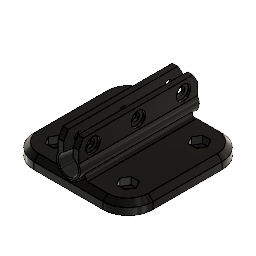
Thermometer Holder v4 (Autodesk Fusion 360 design; units mm, degrees)
Autodesk Fusion 360 part; units mm, degrees
sketch "Sketch1" plane through (0, 0, 0) normal (0, 0, 1) x (1, 0, 0)
  line L0 (-15, 15) -> (15, 15) construction
  line L1 (15, 15) -> (15, -15) construction
  line L2 (15, -15) -> (-15, -15) construction
  line L3 (-15, -15) -> (-15, 15) construction
  line L4 (-15, 15) -> (15, -15) construction
  line L5 (15, 15) -> (-15, -15) construction
  line L6 (25, -25) -> (-25, -25)
  line L7 (-25, -25) -> (-25, 25)
  line L8 (-25, 25) -> (25, 25)
  line L9 (25, 25) -> (25, -25)
  circle A0 centre (15, 15) radius 1.5
  circle A1 centre (-15, 15) radius 1.5
  circle A2 centre (-15, -15) radius 1.5
  circle A3 centre (15, -15) radius 1.5
  circle A4 centre (-15, -15) radius 3
  circle A5 centre (15, -15) radius 3
  circle A6 centre (15, 15) radius 3
  circle A7 centre (-15, 15) radius 3
  line L10 (13.2679, -12) -> (11.5359, -15)
  line L11 (11.5359, -15) -> (13.2679, -18)
  line L12 (13.2679, -18) -> (16.7321, -18)
  line L13 (16.7321, -18) -> (18.4641, -15)
  line L14 (18.4641, -15) -> (16.7321, -12)
  line L15 (16.7321, -12) -> (13.2679, -12)
  line L16 (-16.7321, -12) -> (-18.4641, -15)
  line L17 (-18.4641, -15) -> (-16.7321, -18)
  line L18 (-16.7321, -18) -> (-13.2679, -18)
  line L19 (-13.2679, -18) -> (-11.5359, -15)
  line L20 (-11.5359, -15) -> (-13.2679, -12)
  line L21 (-13.2679, -12) -> (-16.7321, -12)
  line L22 (-16.7321, 18) -> (-18.4641, 15)
  line L23 (-18.4641, 15) -> (-16.7321, 12)
  line L24 (-16.7321, 12) -> (-13.2679, 12)
  line L25 (-13.2679, 12) -> (-11.5359, 15)
  line L26 (-11.5359, 15) -> (-13.2679, 18)
  line L27 (-13.2679, 18) -> (-16.7321, 18)
  line L28 (13.2679, 18) -> (11.5359, 15)
  line L29 (11.5359, 15) -> (13.2679, 12)
  line L30 (13.2679, 12) -> (16.7321, 12)
  line L31 (16.7321, 12) -> (18.4641, 15)
  line L32 (18.4641, 15) -> (16.7321, 18)
  line L33 (16.7321, 18) -> (13.2679, 18)
  point P0 (15, -15)
  point P1 (-15, -15)
  point P2 (-15, 15)
  point P3 (15, 15)
  dimension "d1" = 30
  dimension "d2" = 30
  dimension "d3" = -10
  dimension "d4" = 3
  dimension "d5" = 3
  dimension "d6" = 3
  dimension "d7" = 3
  dimension "d10" = 6
  dimension "d11" = 6
  dimension "d12" = 6
  dimension "d13" = 6
  constraint perpendicular L0 L1
  constraint parallel L0 L2
  constraint parallel L1 L3
  constraint horizontal L0
  constraint coincident L4 origin
  constraint coincident L5 origin
  constraint coincident P3 L0.end
  constraint coincident P2 L0.start
  constraint coincident P1 L2.end
  constraint coincident P0 L1.end
  constraint concentric A1 A7
  measures "d1" distance of L0.end P0
  measures "d2" distance of P0 P1
  measures "d4" diameter of A0
  measures "d5" diameter of A1
  measures "d6" diameter of A2
  measures "d7" diameter of A3
  measures "d10" diameter of A4
  measures "d11" diameter of A5
  measures "d12" diameter of A6
  measures "d13" diameter of A7
extrude "Extrude1" add sketch "Sketch1" along normal blind 5 contours L6 L7 L8 L9
extrude "Extrude2" add sketch "Sketch1" along normal blind 2 contours A4 | A4 L19 L20 | A4 L20 L21 | A4 L18 L19 | A4 L16 L21 | A4 L17 L18 | A4 L16 L17 | A5 | A5 L13 L14 | A5 L14 L15 | A5 L12 L13 | A5 L10 L15 | A5 L11 L12 | A5 L10 L11 | A6 | A6 L31 L32 | A6 L32 L33 | A6 L30 L31 | A6 L28 L33 | A6 L29 L30 | A6 L28 L29 | A7 | A7 L25 L26 | A7 L26 L27 | A7 L24 L25 | A7 L22 L27 | A7 L23 L24 | A7 L22 L23
sketch "Sketch2" plane through (0, -25, 0) normal (0, -1, 0) x (1, 0, 0)
  line L0 (-25, 0) -> (25, 0)
  line L1 (25, 0) -> (25, 5)
  line L2 (25, 5) -> (-25, 5)
  line L3 (-25, 5) -> (-25, 0)
  circle A0 centre (0, 9) radius 3
  circle A1 centre (0, 9) radius 5
  line L4 (0, 12) -> (0, 14)
  line L5 (2, 12) -> (2, 14)
  line L6 (-2, 12) -> (-2, 14)
  line L7 (-2, 12) -> (-2, 11.517)
  line L8 (-2, 11.517) -> (2, 11.517)
  line L9 (2, 11.517) -> (2, 12)
  line L10 (2, 11.517) -> (4.3203, 11.517)
  line L11 (4.3203, 11.517) -> (4.3203, 19)
  line L12 (4.3203, 19) -> (2, 19)
  line L13 (2, 19) -> (2, 14)
  line L14 (-2, 11.517) -> (-4.3203, 11.517)
  line L15 (-4.3203, 11.517) -> (-4.3203, 19)
  line L16 (-4.3203, 19) -> (-2, 19)
  line L17 (-2, 19) -> (-2, 14)
  line L18 (2, 11.517) -> (2, 10.4)
  line L19 (-2, 11.517) -> (-2, 10.6)
  dimension "d16" = 6
  dimension "d17" = 2
  dimension "d18" = 2
  dimension "d19" = -2
  constraint coincident A0 L4.start
  constraint coincident A1 L4.end
  constraint vertical L4
  constraint parallel L6 L7
  constraint perpendicular L5 L8
  constraint perpendicular L8 L9
  constraint coincident A1 L10.end
  constraint perpendicular L9 L10
  constraint perpendicular L10 L11
  constraint perpendicular L11 L12
  constraint perpendicular L12 L13
  constraint coincident A1 L14.end
  constraint perpendicular L7 L14
  constraint perpendicular L12 L15
  constraint perpendicular L6 L16
  constraint perpendicular L16 L17
  constraint perpendicular L8 L18
  constraint perpendicular L8 L19
  measures "d16" diameter of A0
  measures "d18" distance of L4
  measures "d19" distance of L4
extrude "Extrude3" add sketch "Sketch2" against normal up to surface (50 mm away) contours L2 A0 A1 L10 L14 L18 L19 | A1 L6 L15 L16 L17 | A1 L6 L7 L14 | A1 L5 L9 L10 | A1 L5 L11 L12 L13
sketch "Sketch3" plane through (4.3203, 0, 0) normal (1, 0, 0) x (0, 1, 0)
  line L0 (25, 11.517) -> (25, 19)
  line L1 (25, 19) -> (-25, 19)
  line L2 (-25, 19) -> (-25, 11.517)
  line L3 (-25, 11.517) -> (25, 11.517)
  circle A0 centre (0, 15.5) radius 1.5
  circle A1 centre (0, 15.5) radius 3
  circle A2 centre (-19, 15.5) radius 3
  circle A3 centre (-19, 15.5) radius 1.5
  circle A4 centre (19, 15.5) radius 3
  circle A5 centre (19, 15.5) radius 1.5
  dimension "d22" = 3
  dimension "d23" = 6
  dimension "d26" = 19
  dimension "d27" = 0
  constraint concentric A0 A1
  measures "d22" diameter of A0
  measures "d23" diameter of A1
extrude "Extrude4" add 2 faces at (3.5468, 8.3333, 19) (-3.5468, -8.3333, 19) along direction (0, 0, 1) blind 1
extrude "Extrude5" cut sketch "Sketch3" against normal up to surface (8.6405 mm away) contours A0 | A3 | A5
extrude "Extrude6" cut sketch "Sketch3" against normal blind 1 contours A1 | A2 | A4
sketch "Sketch4" plane through (-4.3203, 0, 0) normal (-1, 0, 0) x (0, -1, 0)
  circle A0 centre (19, 15.5) radius 1.5
  circle A1 centre (0, 15.5) radius 1.5
  circle A2 centre (-19, 15.5) radius 1.5
  line L0 (-25, 20) -> (-25, 11.517)
  line L1 (-25, 11.517) -> (25, 11.517)
  line L2 (25, 11.517) -> (25, 20)
  line L3 (25, 20) -> (-25, 20)
  line L4 (17.2679, 18.5) -> (15.5359, 15.5)
  line L5 (15.5359, 15.5) -> (17.2679, 12.5)
  line L6 (17.2679, 12.5) -> (20.7321, 12.5)
  line L7 (20.7321, 12.5) -> (22.4641, 15.5)
  line L8 (22.4641, 15.5) -> (20.7321, 18.5)
  line L9 (20.7321, 18.5) -> (17.2679, 18.5)
  line L10 (-1.7321, 18.5) -> (-3.4641, 15.5)
  line L11 (-3.4641, 15.5) -> (-1.7321, 12.5)
  line L12 (-1.7321, 12.5) -> (1.7321, 12.5)
  line L13 (1.7321, 12.5) -> (3.4641, 15.5)
  line L14 (3.4641, 15.5) -> (1.7321, 18.5)
  line L15 (1.7321, 18.5) -> (-1.7321, 18.5)
  line L16 (-20.7321, 18.5) -> (-22.4641, 15.5)
  line L17 (-22.4641, 15.5) -> (-20.7321, 12.5)
  line L18 (-20.7321, 12.5) -> (-17.2679, 12.5)
  line L19 (-17.2679, 12.5) -> (-15.5359, 15.5)
  line L20 (-15.5359, 15.5) -> (-17.2679, 18.5)
  line L21 (-17.2679, 18.5) -> (-20.7321, 18.5)
  point P0 (19, 15.5)
  point P1 (0, 15.5)
  point P2 (-19, 15.5)
  constraint coincident P0 A0.centre
  constraint coincident P1 A1.centre
  constraint coincident P2 A2.centre
extrude "Extrude7" cut sketch "Sketch4" against normal blind 1 contours L4 L5 L6 L7 L8 L9 | L10 L11 L12 L13 L14 L15 | L16 L17 L18 L19 L20 L21
fillet "Fillet1" radius 10.5 4 edges at (25, -25, 2.5) (25, 25, 2.5) (-25, 25, 2.5) (-25, -25, 2.5)
chamfer "Chamfer1" distance 2 angle 45 10 edges at (-8.75, 25, 5) (-21.9246, 21.9246, 5) (-25, 0, 5) (-21.9246, -21.9246, 5) (-8.75, -25, 5) (8.75, -25, 5) (21.9246, -21.9246, 5) (25, 0, 5) (21.9246, 21.9246, 5) (8.75, 25, 5)
chamfer "Chamfer2" distance 2 angle 60 4 edges at (-3.1601, -25, 20) (3.1601, -25, 20) (-3.1601, 25, 20) (3.1601, 25, 20) measured on face at (-3.5468, -8.3333, 20) measured on face at (3.5468, 8.3333, 20) measured on face at (-3.5468, -8.3333, 20) measured on face at (3.5468, 8.3333, 20)
chamfer "Chamfer3" distance 7 angle 10 2 edges at (0, -25, 6) (0, 25, 6) measured on face at (2.9733, -8.3333, 8.6009) measured on face at (2.9733, -8.3333, 8.6009)
chamfer "Chamfer4" distance 1 angle 45 2 edges at (0, -24, 4) (0, 24, 4)
fillet "Fillet2" radius 1.5 2 edges at (-3, 0, 5) (3, 0, 5)
